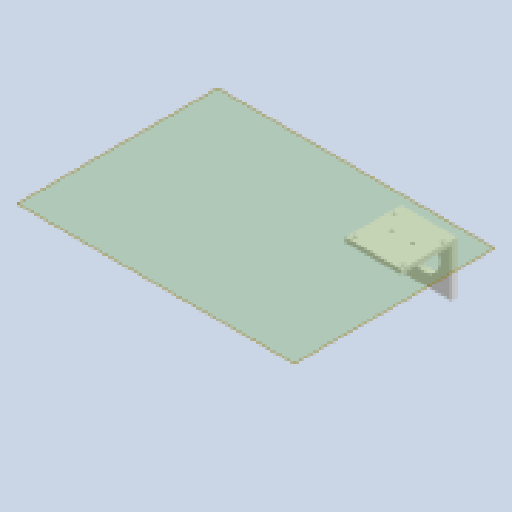
# Autodesk Inventor part: крепление свободной шестерни
Saved by Autodesk Inventor 2024.2 (Build 282272000, 272)
## iProperties
Created: 2025-11-23
Part Number: крепление свободной шестерни
Material: Типовые
Document SubType Name: Modeling
Designer: katya_notebook
Density: 1 g/cm^3
Appearance: По умолчанию
Author: katya_notebook
Autodesk Inventor part; units mm, degrees
ref_plane "YZ Plane" through (0, 0, 0) normal (1, 0, 0) x (0, 1, 0)
ref_plane "XZ Plane" through (0, 0, 0) normal (0, 1, 0) x (-1, 0, 0)
ref_plane "XY Plane" through (0, 0, 0) normal (0, 0, 1) x (1, 0, 0)
ref_plane "РабПлоскость1" through (-232.05, -185.1645, -149.0585) normal (0, -1, 0) x (1, 0, 0)
sketch "Эскиз1" plane through (-232.05, -185.1645, -149.0585) normal (0, -1, 0) x (1, 0, 0)
  line L0 (-135, 97.5) -> (-135, -97.5) projected
  line L1 (-118.5237, -91) -> (-118.5237, -37.5) projected
  line L2 (-135, -79.6587) -> (-135, -55.4979)
  line L3 (-118.5237, -55.4979) -> (-118.5237, -79.6587)
  line L4 (-118.5237, -55.4979) -> (-135, -55.4979)
  line L5 (-0.1223, -79.6587) -> (-0.1223, 72.5986)
  line L6 (118.2792, -55.4979) -> (134.7555, -55.4979)
  line L7 (-118.5237, -97.5) -> (-58.5237, -97.5) projected
  line L8 (118.2792, -97.5) -> (58.2792, -97.5)
  line L9 (58.2792, -97.5) -> (58.2792, -37.5)
  line L10 (58.2792, -37.5) -> (118.2792, -37.5)
  line L11 (118.2792, -37.5) -> (118.2792, -97.5)
  point P0 (232.05, 149.0585)
  point P1 (118.2792, -37.5)
  dimension "d1" = 60
  dimension "d2" = 60
  constraints: 18 end point, 4 point on line, 3 symmetric about line, 2 parallel, 2 perpendicular, 1 horizontal, 1 vertical
  measures "d1" distance of L10.end L8.start
  measures "d2" distance of L9.end L10.end
ref_plane "РабПлоскость2" through (-334.9307, -190.1645, -233.6585) normal (0, 1, 0) x (0, 0, 1)
extrude "Выдавливание1" add sketch "Эскиз1" along normal up to surface (5 mm away)
sketch "Эскиз2" plane through (-173.7708, -190.1645, -186.5585) normal (0, -1, 0) x (1, 0, 0)
  circle A0 centre (-172.803, -47.5) radius 2 projected
  circle A1 centre (-120.803, -47.5) radius 2 projected
  circle A2 centre (-120.803, -5) radius 2 projected
  circle A3 centre (-172.803, -5) radius 2 projected
  line L0 (-193.2792, 135) -> (-193.2792, -60) projected
  line L1 (76.7208, -60) -> (76.7208, 135) projected
  line L2 (-193.2792, -60) -> (-58.2792, -60)
  line L3 (-58.2792, -60) -> (-58.2792, 32.9889)
  circle A4 centre (56.2445, -47.5) radius 2
  circle A5 centre (4.2445, -47.5) radius 2
  circle A6 centre (4.2445, -5) radius 2
  circle A7 centre (56.2445, -5) radius 2
  point P0 (173.7708, 186.5585)
  dimension "d5" = 135
  constraints: 4 centre point, 4 end point, 4 symmetric about line, 1 horizontal, 1 vertical, 4 other
  measures "d5" distance of L0.end L2.end
extrude "Выдавливание2" cut sketch "Эскиз2" against normal blind 10 contours A4 | A5 | A6 | A7
sketch "Эскиз3" plane through (-173.7708, -190.1645, -186.5585) normal (0, -1, 0) x (1, 0, 0)
  line L0 (0, -60) -> (60, -60) projected
  line L1 (0, -60) -> (60, -60)
  line L2 (60, -60) -> (60, -53.5)
  line L3 (60, -53.5) -> (0, -53.5)
  line L4 (0, -53.5) -> (0, -60)
  point P0 (173.7708, 186.5585)
  dimension "d8" = 6.5
  constraints: 8 end point, 2 parallel, 1 horizontal, 1 perpendicular
  measures "d8" distance of L1.end L2.end
sketch "Эскиз4" plane through (-173.7708, -190.1645, -186.5585) normal (0, -1, 0) x (1, 0, 0)
  spline S0 degree 3 poles (43.2445, -30) (43.2445, -30.1203) (43.2336, -30.2387) (43.1929, -30.4661) (43.1631, -30.5751) (43.0528, -30.8816) (42.9505, -31.0587) (42.5833, -31.5484) (42.2402, -31.7817) (41.4641, -32.0292) (41.03, -32.0367) (40.4334, -31.8378) (40.2391, -31.7434) (39.8778, -31.4773) (39.7111, -31.305) (39.4834, -30.9643) (39.3942, -30.7855) (39.2746, -30.4002) (39.2445, -30.1935) (39.2445, -29.8065) (39.2746, -29.5998) (39.3942, -29.2145) (39.4834, -29.0357) (39.7111, -28.695) (39.8778, -28.5227) (40.2391, -28.2566) (40.4334, -28.1622) (41.03, -27.9633) (41.4641, -27.9708) (42.2402, -28.2183) (42.5833, -28.4516) (42.9505, -28.9413) (43.0528, -29.1184) (43.1631, -29.4249) (43.1929, -29.5339) (43.2336, -29.7613) (43.2445, -29.8797) (43.2445, -30) knots 0 0 0 0 0.036086 0.036086 0.072173 0.072173 0.144346 0.144346 0.322747 0.322747 0.501149 0.501149 0.577509 0.577509 0.653869 0.653869 0.711915 0.711915 0.769961 0.769961 0.828007 0.828007 0.886052 0.886052 0.962412 0.962412 1.038772 1.038772 1.217174 1.217174 1.395575 1.395575 1.467748 1.467748 1.503835 1.503835 1.539921 1.539921 1.539921 1.539921 projected
  spline S1 degree 3 poles (20.7277, -30) (20.7277, -30.1752) (20.703, -30.3631) (20.604, -30.7163) (20.53, -30.8816) (20.3402, -31.202) (20.1997, -31.3694) (19.8919, -31.6391) (19.7251, -31.7419) (19.1904, -31.9904) (18.7862, -32.034) (18.0457, -31.9171) (17.7092, -31.7574) (17.2213, -31.3457) (16.9969, -31.0683) (16.8255, -30.6264) (16.7899, -30.5111) (16.7409, -30.2621) (16.7277, -30.1279) (16.7277, -29.8721) (16.7409, -29.7379) (16.7899, -29.4889) (16.8255, -29.3736) (16.9969, -28.9317) (17.2213, -28.6543) (17.7092, -28.2426) (18.0457, -28.0829) (18.7862, -27.966) (19.1904, -28.0096) (19.7251, -28.2581) (19.8919, -28.3609) (20.1997, -28.6306) (20.3402, -28.798) (20.53, -29.1184) (20.604, -29.2837) (20.703, -29.6369) (20.7277, -29.8248) (20.7277, -30) knots 0 0 0 0 0.052568 0.052568 0.105137 0.105137 0.174601 0.174601 0.244066 0.244066 0.414781 0.414781 0.585496 0.585496 0.721852 0.721852 0.760221 0.760221 0.798591 0.798591 0.83696 0.83696 0.875329 0.875329 1.011685 1.011685 1.1824 1.1824 1.353115 1.353115 1.42258 1.42258 1.492044 1.492044 1.544613 1.544613 1.597181 1.597181 1.597181 1.597181 projected
  point P0 (173.7708, 186.5585)
  point P1 (43.2445, -30)
  point P2 (20.7277, -30)
extrude "Выдавливание3" cut sketch "Эскиз4" against normal blind 10
ref_plane "РабПлоскость3" through (-350.5737, -240.8695, -246.5585) normal (0, -1, 0) x (1, 0, 0)
extrude "Выдавливание4" add sketch "Эскиз3" along normal up to surface (50.705 mm away)
sketch "Эскиз5" plane through (-173.7708, -240.8695, -246.5585) normal (0, -1, 0) x (1, 0, 0)
  circle A0 centre (-164.803, 3.25) radius 1.75 projected
  circle A1 centre (-146.803, 3.25) radius 1.75 projected
  circle A2 centre (-128.803, 3.25) radius 1.75 projected
  line L0 (76.7208, 0) -> (-193.2792, 0) projected
  line L1 (-193.2792, 0) -> (-58.2792, 0)
  line L2 (-58.2792, 0) -> (-58.2792, 88.2878)
  circle A3 centre (48.2445, 3.25) radius 1.75
  circle A4 centre (30.2445, 3.25) radius 1.75
  circle A5 centre (12.2445, 3.25) radius 1.75
  point P0 (173.7708, 246.5585)
  dimension "d13" = 135
  constraints: 4 end point, 3 centre point, 3 symmetric about line, 1 midpoint, 1 vertical, 3 other
  measures "d13" distance of L1.end L0.end
ref_plane "РабПлоскость4" through (-340.3237, -230.8695, -245.0585) normal (0, -1, 0) x (1, 0, 0)
extrude "Выдавливание5" cut sketch "Эскиз5" against normal up to surface (10 mm away) contours A3 | A4 | A5
sketch "Эскиз6" plane through (-173.7708, -190.1645, -240.0585) normal (0, 0, 1) x (1, 0, 0)
  circle A0 centre (30.2445, -21) radius 2.5 projected
  circle A1 centre (30.2445, -21) radius 17.5
  point P0 (173.7708, 190.1645)
  dimension "d16" = 35
  constraints: 1 centre point, 1 coincident
  measures "d16" diameter of A1
extrude "Выдавливание6" cut sketch "Эскиз6" against normal blind 10 contours A0 | A1
